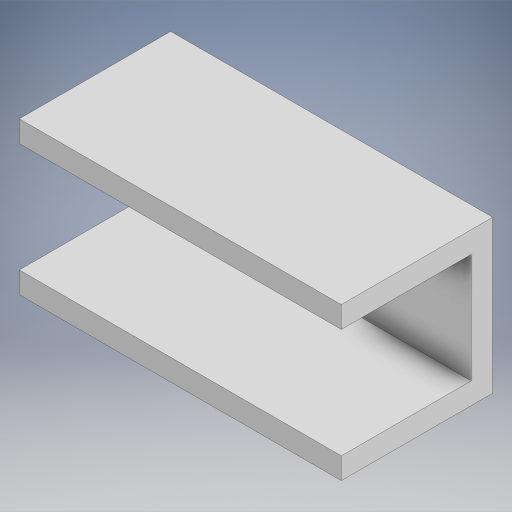
# Autodesk Inventor part: 2024-900-004-REV2
Saved by Autodesk Inventor 2024.2 (Build 282272000, 272)
## iProperties
Created: 2024-03-11
Part Number: 2024-900-004-REV2
Material: Generic
Document SubType Name: Modeling
Designer: rohan
Density: 1 g/cm^3
Appearance: Default
Author: rohan
Autodesk Inventor part; units mm, degrees
ref_plane "YZ Plane" through (0, 0, 0) normal (1, 0, 0) x (0, 1, 0)
ref_plane "XZ Plane" through (0, 0, 0) normal (0, 1, 0) x (-1, 0, 0)
ref_plane "XY Plane" through (0, 0, 0) normal (0, 0, 1) x (1, 0, 0)
sketch "Sketch1" plane through (0, 0, 0) normal (1, 0, 0) x (0, 1, 0)
  line L0 (12.954, 12.7) -> (12.954, -12.954)
  line L1 (12.954, -12.954) -> (-12.954, -12.954)
  line L2 (-12.954, -12.954) -> (-12.954, 12.7)
  line L3 (12.954, 17.78) -> (18.034, 17.78)
  line L4 (18.034, 17.78) -> (18.034, -18.034)
  line L5 (18.034, -18.034) -> (-18.034, -18.034)
  line L6 (-18.034, -18.034) -> (-18.034, 17.78)
  line L7 (-18.034, 17.78) -> (-12.954, 17.78)
  line L8 (12.954, 12.7) -> (12.954, 17.78)
  line L9 (-12.954, 12.7) -> (-12.954, 17.78)
  point P0 (0, 0)
  constraints: 20 end point, 2 parallel, 2 perpendicular, 2 other
extrude "Extrusion1" add sketch "Sketch1" along normal blind 76.2
body "Solid1"
